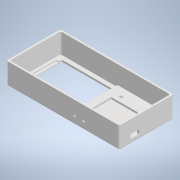
# Autodesk Inventor part: LowerHalf
Saved by Autodesk Inventor 2022 (Build 260153000, 153)
## iProperties
Created: 2023-09-02
Part Number: LowerHalf
Material: Generic
Document SubType Name: Modeling
Designer: Petr Černý
Density: 1 g/cm^3
Appearance: Default
Author: Petr Černý
Autodesk Inventor part; units mm, degrees
ref_plane "YZ Plane" through (0, 0, 0) normal (1, 0, 0) x (0, 1, 0)
ref_plane "XZ Plane" through (0, 0, 0) normal (0, 1, 0) x (-1, 0, 0)
ref_plane "XY Plane" through (0, 0, 0) normal (0, 0, 1) x (1, 0, 0)
sketch "Sketch1" plane through (0, 0, 0) normal (0, 1, 0) x (-1, 0, 0)
  line L0 (-16.8935, 33.2698) -> (108.1065, 33.2698)
  line L1 (108.1065, 33.2698) -> (108.1065, -26.7302)
  line L2 (108.1065, -26.7302) -> (-16.8935, -26.7302)
  line L3 (-16.8935, -26.7302) -> (-16.8935, 33.2698)
  point P0 (0, 0)
  dimension "d0" = 60
  dimension "d1" = 125
  constraints: 8 end point, 2 parallel, 1 horizontal, 1 perpendicular
  measures "d0" distance of L2.end L0.start
  measures "d1" distance of L1.end L2.end
extrude "Extrusion1" add sketch "Sketch1" along normal blind 20
shell "Shell1" thickness 2 removed faces 1 at (-24.7732, 20, -6.7302)
sketch "Sketch2" plane through (-106.1065, 2, -24.7302) normal (0, 1, 0) x (1, 0, 0)
  line L0 (121, 0) -> (121, -56) projected
  line L1 (121, -56) -> (111, -56)
  line L2 (111, -56) -> (111, -46)
  line L3 (111, -46) -> (121, -46)
  line L4 (121, -46) -> (121, -56)
  line L5 (0, 0) -> (121, 0) projected
  line L6 (121, -10) -> (121, 0)
  line L7 (121, -56) -> (0, -56) projected
  line L8 (81, -56) -> (71, -56)
  line L9 (71, -56) -> (71, -46)
  line L10 (71, -46) -> (81, -46)
  line L11 (81, -46) -> (81, -56)
  line L12 (121, 0) -> (71, 0)
  line L13 (71, 0) -> (71, -15)
  line L14 (71, -15) -> (121, -15)
  line L15 (121, -15) -> (121, 0)
  line L16 (71, -56) -> (60.5, -56)
  line L17 (71, 0) -> (71, -56)
  line L18 (71, -56) -> (63, -56)
  line L19 (63, -56) -> (63, 0)
  line L20 (63, 0) -> (71, 0)
  line L21 (71, 0) -> (71, -56)
  point P0 (106.1065, -24.7302)
  point P1 (76, -51.55)
  point P2 (76, -9.45)
  point P3 (116, -9.4)
  point P4 (116, -51.5)
  point P5 (71, -56)
  point P6 (71, -15)
  point P7 (121, -15)
  point P8 (71, -46)
  dimension "d5" = 10
  dimension "d6" = 10
  dimension "d9" = 10
  dimension "d10" = 10
  dimension "d13" = 30
  dimension "d15" = 4.45
  dimension "d16" = 42.1
  dimension "d17" = 40
  dimension "d18" = 5
  dimension "d19" = 42.1
  dimension "d32" = 4.5
  dimension "d81" = 50
  dimension "d82" = 15
  dimension "d83" = 8
  constraints: 38 end point, 8 parallel, 5 horizontal, 4 perpendicular, 2 point on line
  measures "d5" distance of L2.end L3.end
  measures "d6" distance of L1.end L2.end
  measures "d9" distance of L9.end L10.end
  measures "d10" distance of L8.end L9.end
  measures "d13" distance between parallel lines of L11 L2
  measures "d15" distance from line of L8 point (76, -51.55)
  measures "d16" distance of point (76, -9.45) point (76, -51.55)
  measures "d17" distance of point (116, -51.5) point (76, -51.55)
  measures "d18" distance from line of L0 point (116, -51.5)
  measures "d19" distance of point (116, -9.4) point (116, -51.5)
  measures "d32" distance from line of point (116, -51.5) L7
  measures "d81" distance of L14.end L13.end
  measures "d82" distance of L13.end L12.end
  measures "d83" distance of L19.end L20.end
extrude "Extrusion2" add sketch "Sketch2" along normal blind 4 contours L0 L14 L13 L5 | L13 L17 L9 L7 L19 L5 | L0 L1 L2 L3 | L10 L11 L7 L9
sketch "Sketch3" plane through (-106.1065, 6, -24.7302) normal (0, 1, 0) x (1, 0, 0)
  line L0 (123, 2) -> (-2, 2) projected
  line L1 (123, -58) -> (123, 2) projected
  line L2 (-2, -58) -> (123, -58) projected
  line L3 (-2, 2) -> (-2, -58) projected
  point P0 (106.1065, -24.7302)
  point P1 (76, -51.55)
  point P2 (76, -9.45)
  point P3 (116, -9.4)
  point P4 (116, -51.5)
  point P5 (76, -51.55)
  point P6 (76, -9.45)
  point P7 (116, -51.5)
  point P8 (116, -9.4)
  dimension "d29" = 42.1
  dimension "d30" = 42.1
  dimension "d31" = 40
  constraints: 4 coincident
  measures "d29" distance of point (76, -9.45) point (76, -51.55)
  measures "d30" distance of point (116, -9.4) point (116, -51.5)
  measures "d31" distance of point (76, -51.55) point (116, -51.5)
hole "Hole1" at (-30.1065, 6, 26.8198) at (-30.1065, 6, -15.2802) at (9.8935, 6, -15.3302) at (9.8935, 6, 26.7698) direction (0, -1, 0) diameter 3.2 depth 8.8 tip angle 118
sketch "Sketch4" plane through (-108.1065, 0, 33.2698) normal (0, 0, 1) x (1, 0, 0)
  line L0 (72, 16.1171) -> (72, 6.1171) projected
  circle A0 centre (75.47, 8.6194) radius 2.45 projected
  circle A1 centre (85.27, 8.6194) radius 2.45 projected
  circle A2 centre (75.47, 8.6194) radius 2.45
  circle A3 centre (85.27, 8.6194) radius 2.45
  circle A4 centre (86.47, 10.6194) radius 2.45 projected
  circle A5 centre (96.27, 10.6194) radius 2.45 projected
  point P0 (108.1065, 0)
  constraints: 4 coincident, 2 centre point, 2 concentric
hole "Hole2" at (-21.6365, 10.6194, 33.2698) at (-11.8365, 10.6194, 33.2698) direction (0, 0, -1) diameter 2.5 depth 2
sketch "Sketch5" plane through (16.8935, 0, 33.2698) normal (1, 0, 0) x (0, 0, -1)
  line L0 (14, 10.5) -> (23, 10.5)
  line L1 (23, 10.5) -> (23, 7.5)
  line L2 (23, 7.5) -> (14, 7.5)
  line L3 (14, 7.5) -> (14, 10.5)
  line L4 (0, 0) -> (0, 20) projected
  line L5 (0, 0) -> (60, 0) projected
  point P0 (33.2698, 0)
  dimension "d84" = 14
  dimension "d85" = 7.5
  dimension "d86" = 3
  dimension "d87" = 9
  constraints: 8 end point, 2 parallel, 1 horizontal, 1 perpendicular
  measures "d84" distance between parallel lines of L3 L4
  measures "d85" distance between parallel lines of L5 L2
  measures "d86" distance of L0.end L1.end
  measures "d87" distance of L0.start L0.end
extrude "Extrusion3" cut sketch "Sketch5" against normal blind 2
fillet "Fillet1" radius 2 4 edges at (16.8935, 10, 33.2698) (-108.1065, 10, 33.2698) (-108.1065, 10, -26.7302) (16.8935, 10, -26.7302)
fillet "Fillet2" radius 2 4 edges at (-106.1065, 11, -24.7302) (-106.1065, 11, 31.2698) (14.8935, 13, -24.7302) (14.8935, 13, 31.2698)
fillet "Fillet3" radius 2 8 edges at (16.3077, 0, -26.1444) (-45.6065, 0, -26.7302) (-107.5207, 0, -26.1444) (-108.1065, 0, 3.2698) (-107.5207, 0, 32.684) (-45.6065, 0, 33.2698) (16.3077, 0, 32.684) (16.8935, 0, 3.2698)
fillet "Fillet5" radius 1 3 edges at (-25.1065, 4, 21.2698) (-35.1065, 4, 21.2698) (4.8935, 4, 21.2698)
sketch "Sketch7" plane through (0, 0, 0) normal (0, -1, 0) x (1, 0, 0)
  circle A0 centre (9.8935, 26.7698) radius 1.6 projected
  circle A1 centre (9.8935, -15.3302) radius 1.6 projected
  circle A2 centre (-30.1065, 26.8198) radius 1.6 projected
  circle A3 centre (-30.1065, -15.2802) radius 1.6 projected
  point P0 (0, 0)
  constraints: 4 coincident
hole "Hole3" at (9.8935, 0, 26.7698) at (9.8935, 0, -15.3302) at (-30.1065, 0, 26.8198) at (-30.1065, 0, -15.2802) direction (0, 1, 0) diameter 6 depth 3
sketch "Sketch8" plane through (0, 0, 0) normal (0, -1, 0) x (1, 0, 0)
  line L0 (-43.1065, -20.2302) -> (-100.1065, -20.2302)
  line L1 (-100.1065, -20.2302) -> (-100.1065, 26.7698)
  line L2 (-100.1065, 26.7698) -> (-43.1065, 26.7698)
  line L3 (-43.1065, 26.7698) -> (-43.1065, -20.2302)
  line L4 (-108.1065, 31.2698) -> (-108.1065, -24.7302) projected
  line L5 (-106.1065, -26.7302) -> (14.8935, -26.7302) projected
  point P0 (0, 0)
  dimension "d54" = 8
  dimension "d55" = 6.5
  dimension "d56" = 47
  dimension "d57" = 57
  constraints: 8 end point, 2 parallel, 1 horizontal, 1 perpendicular
  measures "d54" distance between parallel lines of L1 L4
  measures "d55" distance between parallel lines of L5 L0
  measures "d56" distance of L2.end L0.start
  measures "d57" distance of L0.start L0.end
extrude "Extrusion4" cut sketch "Sketch8" against normal blind 2
sketch "Sketch11" plane through (0, 0, 0) normal (0, -1, 0) x (1, 0, 0)
  line L0 (-43.1065, -20.2302) -> (-43.1065, 26.7698) projected
  line L1 (-43.1065, 8.2698) -> (-36.1065, 8.2698)
  line L2 (-36.1065, 8.2698) -> (-36.1065, -1.7302)
  line L3 (-36.1065, -1.7302) -> (-43.1065, -1.7302)
  line L4 (-43.1065, -1.7302) -> (-43.1065, 8.2698)
  line L5 (-100.1065, 26.7698) -> (-43.1065, 26.7698) projected
  point P0 (0, 0)
  dimension "d69" = 10
  dimension "d70" = 18.5
  dimension "d71" = 7
  constraints: 8 end point, 2 parallel, 1 horizontal, 1 perpendicular, 1 point on line
  measures "d69" distance of L1.end L2.end
  measures "d70" distance between parallel lines of L5 L1
  measures "d71" distance of L2.end L3.end
extrude "Extrusion7" cut sketch "Sketch11" against normal blind 2
fillet "Fillet7" radius 3 2 edges at (-36.1065, 1, 8.2698) (-36.1065, 1, -1.7302)
sketch "Sketch12" plane through (-106.1065, 2, 29.2698) normal (0, 1, 0) x (1, 0, 0)
  line L0 (6, 2.5) -> (6, 49.5) projected
  line L1 (6, 6) -> (3, 6)
  line L2 (3, 6) -> (3, 46)
  line L3 (3, 46) -> (6, 46)
  line L4 (6, 46) -> (6, 6)
  line L5 (63, 2.5) -> (6, 2.5) projected
  point P0 (106.1065, 29.2698)
  point P1 (6, 46)
  dimension "d75" = 3
  dimension "d76" = 40
  dimension "d77" = 3.5
  constraints: 8 end point, 2 parallel, 1 horizontal, 1 perpendicular, 1 point on line
  measures "d75" distance of L2.end L3.end
  measures "d76" distance of L1.end L2.end
  measures "d77" distance between parallel lines of L1 L5
extrude "Extrusion8" cut sketch "Sketch12" against normal blind 1
fillet "Fillet8" radius 1 2 edges at (-103.1065, 1.5, 23.2698) (-103.1065, 1.5, -16.7302)
body "Solid1"
